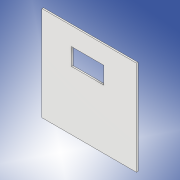
# Autodesk Inventor part: Top Cover
Saved by Autodesk Inventor 2017 SP1 (Build 210196100, 196)
## iProperties
Created: 2017-07-19
Part Number: Top Cover
Material: ABS Plastic
Document SubType Name: Modeling
Designer: zallen
Density: 1.06 g/cm^3
Appearance: CR White
Author: zallen
Autodesk Inventor part; units mm, degrees
ref_plane "YZ Plane" through (0, 0, 0) normal (1, 0, 0) x (0, 1, 0)
ref_plane "XZ Plane" through (0, 0, 0) normal (0, 1, 0) x (-1, 0, 0)
ref_plane "XY Plane" through (0, 0, 0) normal (0, 0, 1) x (1, 0, 0)
sketch "Sketch1" plane through (0, 0, 0) normal (0, 0, 1) x (1, 0, 0)
  line L0 (0, 0) -> (620, 0)
  line L1 (620, 0) -> (620, 620)
  line L2 (620, 620) -> (0, 620)
  line L3 (0, 620) -> (0, 0)
  dimension "d0" = 620
  dimension "d1" = 620
  constraints: 8 end point, 2 parallel, 1 horizontal, 1 perpendicular
  measures "d0" distance of L2.end L1.end
  measures "d1" distance of L1.end L0.end
extrude "Extrusion1" add sketch "Sketch1" along normal blind 10
sketch "Sketch2" plane through (0, 0, 10) normal (0, 0, 1) x (1, 0, 0)
  line L0 (193.5, 388) -> (406.5, 388)
  line L1 (406.5, 388) -> (406.5, 501)
  line L2 (406.5, 501) -> (193.5, 501)
  line L3 (193.5, 501) -> (193.5, 388)
  line L4 (0, 620) -> (0, 0) projected
  line L5 (620, 620) -> (0, 620) projected
  dimension "d4" = 213
  dimension "d5" = 113
  dimension "d6" = 193.5
  dimension "d7" = 119
  constraints: 8 end point, 2 parallel, 1 horizontal, 1 perpendicular
  measures "d4" distance of L2.end L1.end
  measures "d5" distance of L1.end L0.end
  measures "d6" distance between parallel lines of L4 L3
  measures "d7" distance from line of L5 L2.end
extrude "Extrusion2" cut sketch "Sketch2" against normal through all
body "Solid1"
